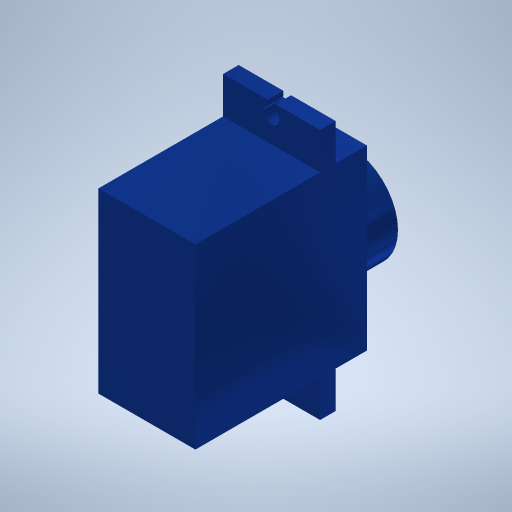
# Autodesk Inventor part: Part8
Saved by Autodesk Inventor 2024 (Build 280153000, 153)
## iProperties
Created: 2017-05-24
Part Number: Part8
Material: PPS Plastic
Document SubType Name: Modeling
Designer: L.Đ.P
Density: 1.637 g/cm^3
Appearance: Smooth - White
Author: L.Đ.P
Autodesk Inventor part; units mm, degrees
ref_plane "YZ Plane" through (0, 0, 0) normal (1, 0, 0) x (0, 1, 0)
ref_plane "XZ Plane" through (0, 0, 0) normal (0, 1, 0) x (-1, 0, 0)
ref_plane "XY Plane" through (0, 0, 0) normal (0, 0, 1) x (1, 0, 0)
sketch "Sketch1" plane through (0, 0, 0) normal (0, 1, 0) x (-1, 0, 0)
  line L0 (6.225, -11.4) -> (-6.225, -11.4)
  line L1 (-6.225, -11.4) -> (-6.225, 11.4)
  line L2 (-6.225, 11.4) -> (6.225, 11.4)
  line L3 (6.225, 11.4) -> (6.225, -11.4)
  line L4 (0, 0) -> (0, -6.7915)
  line L5 (0, 0) -> (-3.4264, 0)
  point P0 (0, -11.4)
  point P1 (-6.225, 0)
  dimension "d0" = 12.45
  dimension "d1" = 22.8
  constraints: 12 end point, 3 parallel, 2 midpoint, 2 perpendicular, 2 point on line, 1 horizontal
  measures "d0" distance of L1.end L2.end
  measures "d1" distance of L0.end L1.end
extrude "Extrusion1" add sketch "Sketch1" along normal blind 16
sketch "Sketch2" plane through (0, 16, 0) normal (0, 1, 0) x (1, 0, 0)
  line L0 (-6.225, 11.4) -> (-6.225, -11.4) projected
  line L1 (6.225, -11.4) -> (6.225, 11.4) projected
  line L2 (6.225, -16.115) -> (-6.225, -16.115)
  line L3 (-6.225, -16.115) -> (-6.225, 16.115)
  line L4 (-6.225, 16.115) -> (6.225, 16.115)
  line L5 (6.225, 16.115) -> (6.225, -16.115)
  point P0 (0, 0)
  point P1 (-6.225, 0)
  point P2 (6.225, 0)
  dimension "d4" = 32.23
  constraints: 8 end point, 4 midpoint, 2 parallel, 1 horizontal, 1 perpendicular
  measures "d4" distance between parallel lines of L2 L4
extrude "Extrusion2" add sketch "Sketch2" along normal blind 2
sketch "Sketch3" plane through (0, 18, 0) normal (0, 1, 0) x (1, 0, 0)
  line L0 (-6.225, 11.4) -> (6.225, 11.4) projected
  line L1 (6.225, 11.4) -> (6.225, -11.4) projected
  line L2 (6.225, -11.4) -> (-6.225, -11.4) projected
  line L3 (-6.225, -11.4) -> (-6.225, 11.4) projected
  line L4 (6.225, -16.115) -> (-6.225, -16.115) projected
  line L5 (-6.225, -16.115) -> (-6.225, 16.115) projected
  line L6 (-6.225, 16.115) -> (6.225, 16.115) projected
  line L7 (6.225, 16.115) -> (6.225, -16.115) projected
  line L8 (6.225, -16.115) -> (-6.225, -16.115) projected
  line L9 (-6.225, -16.115) -> (-6.225, 16.115) projected
  line L10 (-6.225, 16.115) -> (6.225, 16.115) projected
  line L11 (6.225, 16.115) -> (6.225, -16.115) projected
  point P0 (0, 0)
extrude "Extrusion3" add sketch "Sketch3" along normal blind 4 contours L0 L1 L2 L3
sketch "Sketch4" plane through (0, 22, 0) normal (0, 1, 0) x (1, 0, 0)
  line L0 (-6.225, 11.4) -> (-6.225, -11.4) projected
  line L1 (6.225, -11.4) -> (6.225, 11.4) projected
  circle A0 centre (0, 0) radius 6.225
  circle A1 centre (0, 0) radius 1.5
  point P0 (0, 0)
  dimension "d10" = 3
  constraints: 2 centre point, 2 coincident, 2 tangent
  measures "d10" diameter of A1
extrude "Extrusion4" add sketch "Sketch4" along normal blind 4 contours A0 | A1
sketch "Sketch5" plane through (0, 18, 0) normal (0, 1, 0) x (1, 0, 0)
  line L0 (-6.225, -16.115) -> (6.225, -16.115) projected
  line L1 (6.225, -16.115) -> (6.225, -11.4) projected
  circle A0 centre (0, -14.615) radius 1
  line L2 (0.5, -16.115) -> (-0.5, -16.115)
  line L3 (-0.5, -16.115) -> (-0.5, -15.115)
  line L4 (-0.5, -15.115) -> (0.5, -15.115)
  line L5 (0.5, -15.115) -> (0.5, -16.115)
  point P0 (0, 0)
  point P1 (0, -16.115)
  dimension "d15" = 2
  dimension "d16" = 1.5
  dimension "d17" = 1
  dimension "d18" = 1
  dimension "d19" = 6.225
  constraints: 8 end point, 2 midpoint, 2 parallel, 1 centre point, 1 horizontal, 1 perpendicular, 1 point on line
  measures "d15" diameter of A0
  measures "d16" distance from line of L0 A0.centre
  measures "d17" distance of L3.end L4.end
  measures "d18" distance of L2.end L3.end
  measures "d19" distance from line of L1 A0.centre
extrude "Extrusion5" cut sketch "Sketch5" against normal blind 4
mirror "Mirror3" about plane through (0, 0, 0) normal (0, 0, 1) of "Extrusion5"
sketch "Sketch11" plane through (0, 26, 0) normal (0, 1, 0) x (1, 0, 0)
  arc A0 (6.225, 0) -> (6.225, 0) centre (0, 0) ccw projected
  circle A1 centre (0, 0) radius 2.5
  point P0 (0, 0)
  dimension "d49" = 5
  constraints: 1 centre point, 1 coincident
  measures "d49" diameter of A1
extrude "Extrusion11" add sketch "Sketch11" along normal blind 2 contours A1
body "Solid1"
